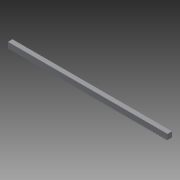
# Autodesk Inventor part: rack
Saved by Autodesk Inventor 2015 SP1 (Build 190203100, 203)
## iProperties
Created: 2015-01-14
Part Number: rack
Material: Generic
Document SubType Name: Modeling
Designer: Jarod
Density: 1 g/cm^3
Appearance: Default
Author: Jarod
Autodesk Inventor part; units mm, degrees
ref_plane "YZ Plane" through (0, 0, 0) normal (1, 0, 0) x (0, 1, 0)
ref_plane "XZ Plane" through (0, 0, 0) normal (0, 1, 0) x (-1, 0, 0)
ref_plane "XY Plane" through (0, 0, 0) normal (0, 0, 1) x (1, 0, 0)
sketch "Sketch1" plane through (0, 0, 0) normal (1, 0, 0) x (0, 1, 0)
  line L0 (0, 0) -> (25.4, 0)
  line L1 (25.4, 0) -> (25.4, -19.05)
  line L2 (25.4, -19.05) -> (0, -19.05)
  line L3 (0, -19.05) -> (0, 0)
  dimension "d0" = 25.4
  dimension "d1" = 19.05
  constraints: 8 end point, 2 parallel, 1 horizontal, 1 perpendicular
  measures "d0" distance of L1.end L2.end
  measures "d1" distance of L0.end L1.end
extrude "Extrusion1" add sketch "Sketch1" along normal blind 685.8
sketch "Sketch2" plane through (0, 0, 0) normal (0, 0, 1) x (1, 0, 0)
  line L0 (0, 0) -> (0, 25.4) projected
  line L1 (0, 0) -> (685.8, 0) projected
  line L2 (685.8, 25.4) -> (685.8, 0) projected
  line L3 (0, 25.4) -> (685.8, 25.4) projected
  line L4 (0, 0) -> (1.5875, 0) construction
  line L5 (1.5875, 0) -> (1.5875, 3.175) construction
  line L6 (1.5875, 3.175) -> (0, 3.175) construction
  line L7 (0, 3.175) -> (0, 0) construction
  line L8 (1.5875, 3.175) -> (3.175, 3.175) construction
  line L9 (3.175, 3.175) -> (3.175, 0) construction
  line L10 (3.175, 0) -> (1.5875, 0) construction
  line L11 (1.5875, 0) -> (1.5875, 3.175) construction
  line L12 (3.175, 3.175) -> (4.7625, 3.175) construction
  line L13 (4.7625, 3.175) -> (4.7625, 0) construction
  line L14 (4.7625, 0) -> (3.175, 0) construction
  line L15 (3.175, 0) -> (3.175, 3.175) construction
  line L16 (0, 3.175) -> (1.5875, 0)
  line L17 (1.5875, 0) -> (3.175, 0)
  line L18 (4.7625, 3.175) -> (6.35, 3.175) construction
  line L19 (6.35, 3.175) -> (6.35, 0) construction
  line L20 (6.35, 0) -> (4.7625, 0) construction
  line L21 (4.7625, 0) -> (4.7625, 3.175) construction
  line L22 (3.175, 0) -> (4.7625, 3.175)
  line L23 (4.7625, 3.175) -> (6.35, 3.175)
  line L24 (6.35, 3.175) -> (6.35, 0)
  line L25 (0, 3.175) -> (0, 0)
  line L26 (0, 0) -> (1.5875, 0)
  line L27 (3.175, 0) -> (6.35, 0)
  dimension "d4" = 1.5875
  dimension "d5" = 3.175
  dimension "d6" = 1.5875
  dimension "d7" = 3.175
  dimension "d8" = 1.5875
  dimension "d9" = 3.175
  dimension "d10" = 1.5875
  dimension "d11" = 3.175
  constraints: 48 end point, 11 equal length, 4 horizontal, 4 perpendicular
  measures "d4" distance of L6.end L5.end
  measures "d5" distance of L5.end L4.end
  measures "d6" distance of L9.end L10.end
  measures "d7" distance of L8.end L9.end
  measures "d8" distance of L13.end L14.end
  measures "d9" distance of L12.end L13.end
  measures "d10" distance of L19.end L20.end
  measures "d11" distance of L18.end L19.end
extrude "Extrusion2" cut sketch "Sketch2" against normal blind 685.8 contours L0 L16 L1 | L22 L23 L24 L1
pattern_linear "Rectangular Pattern1" count 108 spacing 6.35 along (1, 0, 0) of "Extrusion2"
body "Solid1"
